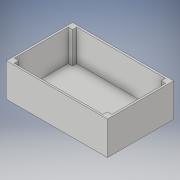
# Autodesk Inventor part: 546-1590J-5.7x3.7-Enclosure
Saved by Autodesk Inventor 2018 (Build 220112000, 112)
## iProperties
Created: 2018-04-27
Part Number: 546-1590J-5.7x3.7-Enclosure
Material: Generic
Document SubType Name: Modeling
Designer: bbramman
Density: 1 g/cm^3
Appearance: Default
Author: bbramman
Autodesk Inventor part; units mm, degrees
ref_plane "YZ Plane" through (0, 0, 0) normal (1, 0, 0) x (0, 1, 0)
ref_plane "XZ Plane" through (0, 0, 0) normal (0, 1, 0) x (-1, 0, 0)
ref_plane "XY Plane" through (0, 0, 0) normal (0, 0, 1) x (1, 0, 0)
sketch "Sketch1" plane through (0, 0, 0) normal (0, 1, 0) x (-1, 0, 0)
  point P0 (0, 0)
sketch "Sketch2" plane through (0, 0, 0) normal (0, 1, 0) x (-1, 0, 0)
  line L0 (-72.5043, 47.2933) -> (72.5043, 47.2933)
  line L1 (72.5043, 47.2933) -> (72.5043, -47.7027)
  line L2 (72.5043, -47.7027) -> (-72.5043, -47.7027)
  line L3 (-72.5043, -47.7027) -> (-72.5043, 47.2933)
  line L4 (-72.5043, 47.2933) -> (72.5043, -47.7027) construction
  line L5 (72.5043, 47.2933) -> (-72.5043, -47.7027) construction
  point P0 (0, 0)
  point P1 (0, -0.2047)
  dimension "d0" = 145.0086
  dimension "d1" = 94.996
  constraints: 12 end point, 2 midpoint, 2 parallel, 1 horizontal, 1 perpendicular
  measures "d0" distance of L1.end L2.end
  measures "d1" distance of L0.end L1.end
extrude "Extrusion1" add sketch "Sketch2" along normal mid plane 2.6924
sketch "Sketch3" plane through (0, 1.3462, 0) normal (0, 1, 0) x (1, 0, 0)
  line L0 (-72.5043, -47.2933) -> (72.5043, -47.2933) projected
  line L1 (72.5043, -47.2933) -> (72.5043, 47.7027) projected
  line L2 (-72.5043, -47.2933) -> (72.5043, -47.2933)
  line L3 (72.5043, -47.2933) -> (72.5043, 47.7027)
  line L4 (72.5043, 47.7027) -> (-72.5043, 47.7027)
  line L5 (-72.5043, 47.7027) -> (-72.5043, -47.2933)
  line L6 (69.8119, -44.8056) -> (-69.8119, 44.8056) construction
  line L7 (-69.8119, -44.8056) -> (69.8119, 44.8056) construction
  line L8 (-72.5043, -47.2933) -> (-63.5127, -47.2933)
  line L9 (-72.5043, -38.3017) -> (-72.5043, -47.2933)
  line L10 (72.5043, 47.7027) -> (-72.5043, 47.7027) projected
  line L11 (-72.5043, 47.7027) -> (-63.5127, 47.7027)
  line L12 (-72.5043, 38.7111) -> (-72.5043, 47.7027)
  line L13 (72.5043, 47.7027) -> (63.5127, 47.7027)
  line L14 (72.5043, 38.7111) -> (72.5043, 47.7027)
  line L15 (72.5043, -47.2933) -> (63.5127, -47.2933)
  line L16 (72.5043, -38.3017) -> (72.5043, -47.2933)
  line L17 (-63.5127, -44.8056) -> (-63.5127, -38.3017)
  line L18 (-63.5127, -38.3017) -> (-69.8119, -38.3017)
  line L19 (-69.8119, 38.7111) -> (-63.5127, 38.7111)
  line L20 (-63.5127, 38.7111) -> (-63.5127, 44.8056)
  line L21 (63.5127, 38.7111) -> (69.8119, 38.7111)
  line L22 (63.5127, 44.8056) -> (63.5127, 38.7111)
  line L23 (63.5127, -44.8056) -> (63.5127, -38.3017)
  line L24 (63.5127, -38.3017) -> (69.8119, -38.3017)
  line L25 (-63.5127, -44.8056) -> (63.5127, -44.8056)
  line L26 (69.8119, -38.3017) -> (69.8119, 38.7111)
  line L27 (63.5127, 44.8056) -> (-63.5127, 44.8056)
  line L28 (-69.8119, 38.7111) -> (-69.8119, -38.3017)
  point P0 (0, 0)
  dimension "d4" = 139.6238
  dimension "d5" = 89.6112
  dimension "d6" = 8.9916
  dimension "d7" = 8.9916
  dimension "d10" = 8.9916
  dimension "d11" = 8.9916
  dimension "d12" = 8.9916
  dimension "d13" = 8.9916
  constraints: 52 end point, 7 horizontal, 6 perpendicular, 2 midpoint, 2 parallel
  measures "d4" distance of L6.end L7.end
  measures "d5" distance of L7.start L6.end
  measures "d6" distance of L9.start L17.end
  measures "d7" distance of L17.end L8.end
  measures "d10" distance of L14.start L21.start
  measures "d11" distance of L21.start L13.end
  measures "d12" distance of L23.end L16.start
  measures "d13" distance of L15.end L23.end
extrude "Extrusion2" add sketch "Sketch3" along normal blind 45.1104
body "Solid1"
